Autodesk Fusion 360 part; units mm, degrees
note: some values were not read from the file. Chosen so that the rebuilt part matches the saved one: which pieces of a blend or face edit are solid. Set by a fixed rule: which sketch regions a step uses.
(part 3 of 3)
  spline S271 degree 3 poles (76.9459, -1.2857) (76.9874, -1.1697) (77.0261, -1.0528) (77.0796, -0.8969) knots 0 0 0 0 1 1 1 1
  line L24 (77.0796, -0.8969) -> (71.8772, -0.8969)
  spline S272 degree 3 poles (71.8772, -0.8969) (71.8728, -0.8474) (71.8656, -0.8253) (71.87, -0.8059) knots 0 0 0 0 1 1 1 1
  spline S273 degree 2 poles (71.87, -0.8059) (72.0386, -0.0634) (72.7928, -0.0634) knots 0 0 0 1 1 1
  spline S274 degree 3 poles (72.7928, -0.0634) (75.5433, -0.0634) (78.2938, -0.0634) (81.0442, -0.0634) knots 0 0 0 0 1 1 1 1
  line L25 (81.0442, -0.0634) -> (81.4689, -0.0634)
  spline S275 degree 3 poles (81.4689, -0.0634) (81.3172, -0.5003) (81.1791, -0.9064) (81.0355, -1.3105) knots 0 0 0 0 1 1 1 1
  spline S276 degree 3 poles (81.0355, -1.3105) (76.5089, -14.0458) (71.9791, -26.78) (67.4605, -39.5181) knots 0 0 0 0 1 1 1 1
  spline S277 degree 3 poles (67.4605, -39.5181) (67.1403, -40.4209) (66.8922, -41.3499) (66.6319, -42.2727) knots 0 0 0 0 1 1 1 1
  spline S278 degree 3 poles (66.6319, -42.2727) (66.5643, -42.5124) (66.5592, -42.7745) (66.5563, -43.0267) knots 0 0 0 0 1 1 1 1
  spline S279 degree 3 poles (66.5563, -43.0267) (66.5417, -44.2641) (67.3792, -44.9721) (68.5993, -44.764) knots 0 0 0 0 1 1 1 1
  spline S280 degree 3 poles (68.5993, -44.764) (69.1748, -44.6659) (69.6796, -44.4126) (70.1463, -44.0705) knots 0 0 0 0 1 1 1 1
  spline S281 degree 3 poles (70.1463, -44.0705) (71.6905, -42.9385) (72.8455, -41.4761) (73.6418, -39.7556) knots 0 0 0 0 1 1 1 1
  spline S282 degree 3 poles (73.6418, -39.7556) (74.1085, -38.7475) (74.4293, -37.6709) (74.7999, -36.6195) knots 0 0 0 0 1 1 1 1
  spline S283 degree 3 poles (74.7999, -36.6195) (76.6624, -31.3356) (78.5196, -26.0499) (80.3787, -20.7648) knots 0 0 0 0 1 1 1 1
  spline S284 degree 3 poles (80.3787, -20.7648) (80.4133, -20.6665) (80.4479, -20.5681) (80.4962, -20.4306) knots 0 0 0 0 1 1 1 1
  line L26 (80.4962, -20.4306) -> (75.2552, -20.4306)
  spline S285 degree 3 poles (75.2552, -20.4306) (75.3359, -20.148) (75.3825, -19.9022) (75.4831, -19.6808) knots 0 0 0 0 1 1 1 1
  spline S286 degree 3 poles (75.4831, -19.6808) (75.5151, -19.6102) (75.6902, -19.574) (75.8, -19.5737) knots 0 0 0 0 1 1 1 1
  spline S287 degree 3 poles (75.8, -19.5737) (77.8099, -19.5675) (79.8199, -19.5691) (81.8299, -19.5691) knots 0 0 0 0 1 1 1 1
  spline S288 degree 3 poles (81.8299, -19.5691) (82.7185, -19.5691) (83.6071, -19.5691) (84.4957, -19.5691) knots 0 0 0 0 1 1 1 1
  line L27 (84.4957, -19.5691) -> (84.8908, -19.5691)
  spline S289 degree 3 poles (84.8908, -19.5691) (84.6969, -20.1342) (84.5194, -20.6587) (84.3372, -21.1815) knots 0 0 0 0 1 1 1 1
  spline S290 degree 3 poles (84.3372, -21.1815) (82.1946, -27.3287) (80.0448, -33.4733) (77.9153, -39.625) knots 0 0 0 0 1 1 1 1
  spline S291 degree 3 poles (77.9153, -39.625) (77.5918, -40.5594) (77.343, -41.5214) (77.099, -42.4806) knots 0 0 0 0 1 1 1 1
  spline S292 degree 3 poles (77.099, -42.4806) (77.0232, -42.7789) (77.0352, -43.1161) (77.0794, -43.4251) knots 0 0 0 0 1 1 1 1
  spline S293 degree 3 poles (77.0794, -43.4251) (77.2211, -44.4149) (78.0389, -44.9766) (79.081, -44.7494) knots 0 0 0 0 1 1 1 1
  spline S294 degree 3 poles (79.081, -44.7494) (79.5647, -44.644) (80.0606, -44.4492) (80.4698, -44.1743) knots 0 0 0 0 1 1 1 1
  spline S295 degree 3 poles (80.4698, -44.1743) (81.9568, -43.1756) (83.0471, -41.8112) (83.893, -40.2456) knots 0 0 0 0 1 1 1 1
  spline S296 degree 3 poles (83.893, -40.2456) (83.9344, -40.169) (83.9365, -40.0409) (83.9031, -39.9585) knots 0 0 0 0 1 1 1 1
  spline S297 degree 3 poles (83.9031, -39.9585) (82.6174, -36.7855) (82.7766, -33.5787) (83.9322, -30.4535) knots 0 0 0 0 1 1 1 1
  spline S298 degree 3 poles (83.9322, -30.4535) (85.9017, -25.1273) (89.5691, -21.403) (94.9427, -19.4482) knots 0 0 0 0 1 1 1 1
  spline S299 degree 3 poles (94.9427, -19.4482) (96.8678, -18.7478) (98.865, -18.5551) (100.8691, -19.0689) knots 0 0 0 0 1 1 1 1
  spline S300 degree 3 poles (100.8691, -19.0689) (103.3851, -19.714) (105.1687, -21.313) (106.3628, -23.5722) knots 0 0 0 0 1 1 1 1
  spline S301 degree 3 poles (106.3628, -23.5722) (107.5188, -25.7593) (107.8486, -28.1077) (107.5537, -30.5511) knots 0 0 0 0 1 1 1 1
  spline S302 degree 3 poles (107.5537, -30.5511) (107.0753, -34.5158) (105.1593, -37.7643) (102.4686, -40.6044) knots 0 0 0 0 1 1 1 1
  spline S303 degree 3 poles (102.4686, -40.6044) (100.6012, -42.5754) (98.3827, -44.0429) (95.8081, -44.9372) knots 0 0 0 0 1 1 1 1
  spline S304 degree 3 poles (95.8081, -44.9372) (93.5986, -45.7048) (91.3614, -45.8636) (89.1334, -45.0354) knots 0 0 0 0 1 1 1 1
  spline S305 degree 3 poles (89.1334, -45.0354) (87.2073, -44.3196) (85.7144, -43.047) (84.6127, -41.3152) knots 0 0 0 0 1 1 1 1
  spline S306 degree 3 poles (84.6127, -41.3152) (84.5617, -41.2351) (84.5132, -41.1534) (84.4605, -41.0746) knots 0 0 0 0 1 1 1 1
  spline S307 degree 3 poles (84.4605, -41.0746) (84.4504, -41.0594) (84.4258, -41.054) (84.4744, -41.0809) knots 0 0 0 0 1 1 1 1
  spline S308 degree 3 poles (84.4744, -41.0809) (83.8997, -41.8316) (83.3916, -42.6279) (82.7546, -43.3024) knots 0 0 0 0 1 1 1 1
  spline S309 degree 3 poles (82.7546, -43.3024) (80.844, -45.3252) (78.4925, -45.9992) (75.7898, -45.3455) knots 0 0 0 0 1 1 1 1
  spline S310 degree 3 poles (75.7898, -45.3455) (74.2035, -44.9618) (73.427, -43.9443) (73.377, -42.3173) knots 0 0 0 0 1 1 1 1
  spline S311 degree 3 poles (73.377, -42.3173) (73.3743, -42.2262) (73.3767, -42.1348) (73.3767, -41.9795) knots 0 0 0 0 1 1 1 1
  spline S312 degree 3 poles (73.3767, -41.9795) (73.0458, -42.3875) (72.7758, -42.7603) (72.4656, -43.096) knots 0 0 0 0 1 1 1 1
  spline S313 degree 3 poles (72.4656, -43.096) (71.2784, -44.3806) (69.8832, -45.31) (68.0996, -45.5148) knots 0 0 0 0 1 1 1 1
  spline S314 degree 3 poles (68.0996, -45.5148) (67.0306, -45.6375) (65.9669, -45.6042) (64.9382, -45.2356) knots 0 0 0 0 1 1 1 1
  spline S315 degree 3 poles (64.9382, -45.2356) (63.5857, -44.7511) (62.923, -43.8262) (62.8928, -42.3877) knots 0 0 0 0 1 1 1 1
  spline S316 degree 3 poles (62.8928, -42.3877) (62.8902, -42.2662) (62.8925, -42.1445) (62.8925, -41.9728) knots 0 0 0 0 1 1 1 1
  spline S317 degree 3 poles (62.8925, -41.9728) (62.5336, -42.4076) (62.2327, -42.813) (61.8902, -43.1798) knots 0 0 0 0 1 1 1 1
  spline S318 degree 3 poles (61.8902, -43.1798) (60.4964, -44.6726) (58.821, -45.5971) (56.731, -45.5649) knots 0 0 0 0 1 1 1 1
  spline S319 degree 3 poles (56.731, -45.5649) (56.0409, -45.5543) (55.3375, -45.4608) (54.6679, -45.2941) knots 0 0 0 0 1 1 1 1
  spline S320 degree 3 poles (54.6679, -45.2941) (53.5786, -45.0228) (53.0763, -44.5495) (52.6072, -43.5745) knots 0 0 0 0 1 1 1 1
  spline S321 degree 3 poles (52.6072, -43.5745) (52.0194, -43.9749) (51.4482, -44.4101) (50.8342, -44.773) knots 0 0 0 0 1 1 1 1
  spline S322 degree 3 poles (50.8342, -44.773) (49.3654, -45.6409) (47.775, -45.7703) (46.1469, -45.3786) knots 0 0 0 0 1 1 1 1
  spline S323 degree 3 poles (46.1469, -45.3786) (44.7538, -45.0434) (43.9596, -44.0239) (43.8607, -42.5731) knots 0 0 0 0 1 1 1 1
  spline S324 degree 3 poles (43.8607, -42.5731) (43.7805, -41.3953) (44.0412, -40.2656) (44.3478, -39.1425) knots 0 0 0 0 1 1 1 1
  spline S325 degree 3 poles (44.3478, -39.1425) (44.3802, -39.0239) (44.4122, -38.9052) (44.3822, -38.747) knots 0 0 0 0 1 1 1 1
  spline S326 degree 3 poles (44.3822, -38.747) (44.2975, -38.8447) (44.2114, -38.9412) (44.1283, -39.0402) knots 0 0 0 0 1 1 1 1
  spline S327 degree 3 poles (44.1283, -39.0402) (42.8844, -40.5225) (41.6555, -42.0196) (40.0946, -43.1941) knots 0 0 0 0 1 1 1 1
  spline S328 degree 3 poles (40.0946, -43.1941) (38.6342, -44.293) (37.0632, -45.1607) (35.2298, -45.4504) knots 0 0 0 0 1 1 1 1
  spline S329 degree 3 poles (35.2298, -45.4504) (33.7641, -45.6821) (32.3176, -45.6378) (30.9433, -45.0022) knots 0 0 0 0 1 1 1 1
  spline S330 degree 3 poles (30.9433, -45.0022) (29.1176, -44.1579) (28.0823, -42.6659) (27.6348, -40.7633) knots 0 0 0 0 1 1 1 1
  spline S331 degree 3 poles (27.6348, -40.7633) (27.443, -39.948) (27.4212, -39.0926) (27.3272, -38.2549) knots 0 0 0 0 1 1 1 1
  spline S332 degree 3 poles (27.3272, -38.2549) (27.3127, -38.1253) (27.3252, -37.9926) (27.2528, -37.8437) knots 0 0 0 0 1 1 1 1
  spline S333 degree 3 poles (27.2528, -37.8437) (27.118, -38.0638) (26.9879, -38.287) (26.8476, -38.5034) knots 0 0 0 0 1 1 1 1
  spline S334 degree 3 poles (26.8476, -38.5034) (24.8612, -41.5667) (22.1611, -43.7524) (18.7272, -44.9928) knots 0 0 0 0 1 1 1 1
  spline S335 degree 3 poles (18.7272, -44.9928) (16.8655, -45.6654) (14.9147, -45.7043) (12.9615, -45.5794) knots 0 0 0 0 1 1 1 1
  spline S336 degree 3 poles (12.9615, -45.5794) (11.4556, -45.483) (9.982, -45.2081) (8.5868, -44.6156) knots 0 0 0 0 1 1 1 1
  spline S337 degree 3 poles (8.5868, -44.6156) (5.0699, -43.1219) (2.7269, -40.5128) (1.4018, -36.9651) knots 0 0 0 0 1 1 1 1
  spline S338 degree 3 poles (1.4018, -36.9651) (0.5889, -34.789) (0.2461, -32.5189) (0.1152, -30.2088) knots 0 0 0 0 1 1 1 1
  spline S339 degree 3 poles (0.1152, -30.2088) (-0.1988, -24.667) (1.4603, -19.6798) (4.4487, -15.0988) knots 0 0 0 0 1 1 1 1
  spline S340 degree 3 poles (4.4487, -15.0988) (7.6391, -10.2081) (11.8716, -6.4708) (17.171, -3.9759) knots 0 0 0 0 1 1 1 1
  spline S341 degree 3 poles (17.171, -3.9759) (18.9174, -3.1537) (20.7361, -2.5457) (22.6573, -2.2749) knots 0 0 0 0 1 1 1 1
  spline S342 degree 3 poles (22.6573, -2.2749) (25.2538, -1.9088) (27.7778, -2.2096) (30.2365, -3.0973) knots 0 0 0 0 1 1 1 1
  spline S343 degree 3 poles (30.2365, -3.0973) (31.1101, -3.4127) (31.9675, -3.7753) (32.8488, -4.0666) knots 0 0 0 0 1 1 1 1
  spline S344 degree 3 poles (32.8488, -4.0666) (33.3657, -4.2376) (33.9099, -4.3637) (34.4509, -4.4166) knots 0 0 0 0 1 1 1 1
  spline S345 degree 3 poles (34.4509, -4.4166) (35.5622, -4.5251) (36.3629, -3.9783) (36.9084, -3.0554) knots 0 0 0 0 1 1 1 1
  spline S346 degree 3 poles (36.9084, -3.0554) (37.0752, -2.7732) (37.2322, -2.6868) (37.5281, -2.7909) knots 0 0 0 0 1 1 1 1
  spline S347 degree 3 poles (37.5281, -2.7909) (37.6735, -2.8421) (37.8301, -2.8615) (38.014, -2.9026) knots 0 0 0 0 1 1 1 1
  spline S348 degree 3 poles (38.014, -2.9026) (37.7215, -3.721) (37.4387, -4.513) (37.1555, -5.3048) knots 0 0 0 0 1 1 1 1
  spline S349 degree 3 poles (37.1555, -5.3048) (36.1535, -8.1065) (35.1509, -10.908) (34.1497, -13.71) knots 0 0 0 0 1 1 1 1
  spline S350 degree 3 poles (34.1497, -13.71) (33.9218, -14.3478) (33.924, -14.3486) (33.1894, -14.2539) knots 0 0 0 0 1 1 1 1
  spline S351 degree 3 poles (33.1894, -14.2539) (33.2661, -13.6185) (33.3592, -12.9843) (33.4161, -12.3467) knots 0 0 0 0 1 1 1 1
  spline S352 degree 3 poles (33.4161, -12.3467) (33.5354, -11.0084) (33.6343, -9.6642) (33.2979, -8.3429) knots 0 0 0 0 1 1 1 1
  spline S353 degree 3 poles (33.2979, -8.3429) (32.7503, -6.1919) (31.4072, -4.6744) (29.3636, -3.8873) knots 0 0 0 0 1 1 1 1
  spline S354 degree 3 poles (29.3636, -3.8873) (25.4024, -2.3618) (21.6115, -2.5974) (18.1064, -5.2075) knots 0 0 0 0 1 1 1 1
  spline S355 degree 3 poles (18.1064, -5.2075) (15.5983, -7.0752) (13.6497, -9.4342) (12.0128, -12.064) knots 0 0 0 0 1 1 1 1
  spline S356 degree 3 poles (12.0128, -12.064) (9.4965, -16.1067) (7.7161, -20.4766) (6.3534, -25.0241) knots 0 0 0 0 1 1 1 1
  spline S357 degree 3 poles (6.3534, -25.0241) (5.5761, -27.6183) (5.0135, -30.2599) (4.7229, -32.9543) knots 0 0 0 0 1 1 1 1
  spline S358 degree 3 poles (4.7229, -32.9543) (4.5192, -34.842) (4.4781, -36.7259) (4.9304, -38.5933) knots 0 0 0 0 1 1 1 1
  spline S359 degree 3 poles (4.9304, -38.5933) (5.6053, -41.3794) (7.3021, -43.2695) (10.0108, -44.1478) knots 0 0 0 0 1 1 1 1
  spline S360 degree 3 poles (10.0108, -44.1478) (13.1649, -45.1705) (16.3359, -45.2186) (19.4152, -43.8207) knots 0 0 0 0 1 1 1 1
  spline S361 degree 3 poles (19.4152, -43.8207) (22.1935, -42.5594) (24.3784, -40.5957) (26.0144, -38.024) knots 0 0 0 0 1 1 1 1
  spline S362 degree 3 poles (26.0144, -38.024) (26.4452, -37.3469) (26.7981, -36.6105) (27.2978, -35.9909) knots 0 0 0 0 1 1 1 1
  spline S363 degree 3 poles (27.2978, -35.9909) (27.6013, -35.6146) (27.6548, -35.2071) (27.7761, -34.8009) knots 0 0 0 0 1 1 1 1
  spline S364 degree 3 poles (27.7761, -34.8009) (28.5607, -32.172) (29.8681, -29.8167) (31.5841, -27.6967) knots 0 0 0 0 1 1 1 1
  spline S365 degree 3 poles (31.5841, -27.6967) (34.2471, -24.4068) (37.4617, -21.785) (41.2974, -19.9603) knots 0 0 0 0 1 1 1 1
  spline S366 degree 3 poles (41.2974, -19.9603) (42.5718, -19.3541) (43.9034, -18.9073) (45.3289, -18.8182) knots 0 0 0 0 1 1 1 1
  spline S367 degree 3 poles (45.3289, -18.8182) (46.5961, -18.7389) (47.768, -19.0007) (48.7702, -19.8267) knots 0 0 0 0 1 1 1 1
  spline S368 degree 3 poles (48.7702, -19.8267) (49.4912, -20.4209) (49.8984, -21.1818) (49.9641, -22.1189) knots 0 0 0 0 1 1 1 1
  spline S369 degree 3 poles (49.9641, -22.1189) (49.9692, -22.1925) (49.9778, -22.2661) (49.9884, -22.3391) knots 0 0 0 0 1 1 1 1
  spline S370 degree 3 poles (49.9884, -22.3391) (49.9927, -22.3689) (50.0063, -22.3974) (50.0157, -22.4264) knots 0 0 0 0 1 1 1 1
  spline S371 degree 3 poles (50.0157, -22.4264) (50.0388, -22.4327) (50.0618, -22.439) (50.0849, -22.4264) knots 0 0 0 0 1 1 1 1
  spline S372 degree 3 poles (103.7652, -25.3114) (103.6868, -24.832) (103.6099, -23.932) (103.3842, -23.071) knots 0 0 0 0 1 1 1 1
  spline S373 degree 3 poles (103.3842, -23.071) (102.9323, -21.3472) (101.8898, -20.1667) (100.0685, -19.7927) knots 0 0 0 0 1 1 1 1
  spline S374 degree 3 poles (100.0685, -19.7927) (97.9906, -19.366) (96.1141, -19.7496) (94.434, -21.0869) knots 0 0 0 0 1 1 1 1
  spline S375 degree 3 poles (94.434, -21.0869) (92.8843, -22.3203) (91.7133, -23.8561) (90.75, -25.561) knots 0 0 0 0 1 1 1 1
  spline S376 degree 3 poles (90.75, -25.561) (88.9387, -28.7669) (87.8127, -32.2136) (87.2249, -35.8387) knots 0 0 0 0 1 1 1 1
  spline S377 degree 3 poles (87.2249, -35.8387) (86.9707, -37.4063) (86.8196, -38.9843) (87.089, -40.569) knots 0 0 0 0 1 1 1 1
  spline S378 degree 3 poles (87.089, -40.569) (87.4308, -42.5797) (88.511, -43.9928) (90.5089, -44.5579) knots 0 0 0 0 1 1 1 1
  spline S379 degree 3 poles (90.5089, -44.5579) (92.2381, -45.047) (93.88, -44.7412) (95.3927, -43.7705) knots 0 0 0 0 1 1 1 1
  spline S380 degree 3 poles (95.3927, -43.7705) (96.8708, -42.822) (98.0012, -41.534) (98.9616, -40.0853) knots 0 0 0 0 1 1 1 1
  spline S381 degree 3 poles (98.9616, -40.0853) (100.7237, -37.4275) (101.8987, -34.5089) (102.7607, -31.4561) knots 0 0 0 0 1 1 1 1
  spline S382 degree 3 poles (102.7607, -31.4561) (103.2897, -29.5826) (103.6858, -27.6833) (103.7652, -25.3114) knots 0 0 0 0 1 1 1 1
  spline S383 degree 3 poles (46.0065, -19.6332) (44.9669, -19.627) (44.0162, -19.8508) (43.1126, -20.2652) knots 0 0 0 0 1 1 1 1
  spline S384 degree 3 poles (43.1126, -20.2652) (41.2513, -21.1186) (39.7466, -22.4329) (38.4102, -23.9545) knots 0 0 0 0 1 1 1 1
  spline S385 degree 3 poles (38.4102, -23.9545) (36.618, -25.9951) (35.2451, -28.3068) (34.0956, -30.753) knots 0 0 0 0 1 1 1 1
  spline S386 degree 3 poles (34.0956, -30.753) (32.774, -33.5658) (31.7466, -36.4734) (31.4534, -39.5941) knots 0 0 0 0 1 1 1 1
  spline S387 degree 3 poles (31.4534, -39.5941) (31.3429, -40.7711) (31.3958, -41.9355) (31.8603, -43.0504) knots 0 0 0 0 1 1 1 1
  spline S388 degree 3 poles (31.8603, -43.0504) (32.3368, -44.1941) (33.2068, -44.7345) (34.4271, -44.7672) knots 0 0 0 0 1 1 1 1
  spline S389 degree 3 poles (34.4271, -44.7672) (35.6477, -44.7998) (36.7623, -44.4442) (37.8098, -43.852) knots 0 0 0 0 1 1 1 1
  spline S390 degree 3 poles (37.8098, -43.852) (40.0373, -42.5928) (41.8175, -40.8319) (43.3761, -38.8332) knots 0 0 0 0 1 1 1 1
  spline S391 degree 3 poles (43.3761, -38.8332) (44.1228, -37.8756) (44.8434, -36.8973) (45.2618, -35.7354) knots 0 0 0 0 1 1 1 1
  spline S392 degree 3 poles (45.2618, -35.7354) (46.3267, -32.778) (47.4017, -29.8244) (48.4649, -26.8664) knots 0 0 0 0 1 1 1 1
  spline S393 degree 3 poles (48.4649, -26.8664) (48.8497, -25.7959) (49.3037, -24.7413) (49.4107, -23.5928) knots 0 0 0 0 1 1 1 1
  spline S394 degree 3 poles (49.4107, -23.5928) (49.6232, -21.3105) (48.1691, -19.514) (46.0065, -19.6332) knots 0 0 0 0 1 1 1 1
  spline S395 degree 3 poles (84.1667, -10.1913) (84.1729, -8.6259) (85.3768, -7.4326) (86.9503, -7.4324) knots 0 0 0 0 1 1 1 1
  spline S396 degree 3 poles (86.9503, -7.4324) (88.5314, -7.4321) (89.7239, -8.6369) (89.7211, -10.2316) knots 0 0 0 0 1 1 1 1
  spline S397 degree 3 poles (89.7211, -10.2316) (89.7183, -11.8206) (88.5136, -13.0149) (86.9258, -13.0029) knots 0 0 0 0 1 1 1 1
  spline S398 degree 3 poles (86.9258, -13.0029) (85.3374, -12.9908) (84.1605, -11.7915) (84.1667, -10.1913) knots 0 0 0 0 1 1 1 1
  spline S399 degree 3 poles (128.8614, -26.1716) (128.8153, -28.284) (128.276, -30.6235) (127.5153, -32.9166) knots 0 0 0 0 1 1 1 1
  spline S400 degree 3 poles (127.5153, -32.9166) (126.5931, -35.6965) (125.3817, -38.3368) (123.61, -40.6911) knots 0 0 0 0 1 1 1 1
  spline S401 degree 3 poles (123.61, -40.6911) (122.5647, -42.0801) (121.3489, -43.2903) (119.806, -44.129) knots 0 0 0 0 1 1 1 1
  spline S402 degree 3 poles (119.806, -44.129) (118.0331, -45.0928) (115.4801, -45.0947) (113.845, -43.5861) knots 0 0 0 0 1 1 1 1
  spline S403 degree 3 poles (113.845, -43.5861) (112.9324, -42.7442) (112.3341, -41.7221) (111.9863, -40.5443) knots 0 0 0 0 1 1 1 1
  spline S404 degree 3 poles (111.9863, -40.5443) (111.834, -40.0287) (111.687, -39.5095) (111.5818, -38.983) knots 0 0 0 0 1 1 1 1
  spline S405 degree 3 poles (111.5818, -38.983) (111.5353, -38.7499) (111.5424, -38.4751) (111.6206, -38.2527) knots 0 0 0 0 1 1 1 1
  spline S406 degree 3 poles (111.6206, -38.2527) (113.0797, -34.1034) (114.5515, -29.9585) (116.0281, -25.8153) knots 0 0 0 0 1 1 1 1
  spline S407 degree 3 poles (116.0281, -25.8153) (116.1079, -25.5914) (116.2291, -25.3728) (116.3717, -25.182) knots 0 0 0 0 1 1 1 1
  spline S408 degree 3 poles (116.3717, -25.182) (117.2705, -23.9794) (118.185, -22.7878) (119.3159, -21.7871) knots 0 0 0 0 1 1 1 1
  spline S409 degree 3 poles (119.3159, -21.7871) (120.4047, -20.8235) (121.5941, -20.0336) (123.056, -19.7578) knots 0 0 0 0 1 1 1 1
  spline S410 degree 3 poles (123.056, -19.7578) (123.9276, -19.5934) (124.8028, -19.5937) (125.6676, -19.8061) knots 0 0 0 0 1 1 1 1
  spline S411 degree 3 poles (125.6676, -19.8061) (126.9085, -20.111) (127.6838, -20.9266) (128.1613, -22.0809) knots 0 0 0 0 1 1 1 1
  spline S412 degree 3 poles (128.1613, -22.0809) (128.6621, -23.2915) (128.8638, -24.5521) (128.8614, -26.1716) knots 0 0 0 0 1 1 1 1
  spline S413 degree 3 poles (138.7712, -30.0038) (139.2283, -29.0291) (139.6235, -28.0968) (140.0927, -27.2034) knots 0 0 0 0 1 1 1 1
  spline S414 degree 3 poles (140.0927, -27.2034) (141.2378, -25.0227) (142.6739, -23.0631) (144.619, -21.5155) knots 0 0 0 0 1 1 1 1
  spline S415 degree 3 poles (144.619, -21.5155) (145.6449, -20.6992) (146.7387, -19.9808) (148.0608, -19.7806) knots 0 0 0 0 1 1 1 1
  spline S416 degree 3 poles (148.0608, -19.7806) (148.7512, -19.6761) (149.4761, -19.6581) (150.1687, -19.7408) knots 0 0 0 0 1 1 1 1
  spline S417 degree 3 poles (150.1687, -19.7408) (151.3327, -19.8797) (152.1161, -20.7367) (152.2726, -21.9102) knots 0 0 0 0 1 1 1 1
  spline S418 degree 3 poles (152.2726, -21.9102) (152.4727, -23.4101) (151.9809, -24.7224) (151.122, -25.9174) knots 0 0 0 0 1 1 1 1
  spline S419 degree 3 poles (151.122, -25.9174) (149.935, -27.569) (148.2949, -28.6145) (146.4395, -29.3662) knots 0 0 0 0 1 1 1 1
  spline S420 degree 3 poles (146.4395, -29.3662) (144.4026, -30.1915) (142.2832, -30.356) (140.1191, -30.1628) knots 0 0 0 0 1 1 1 1
  spline S421 degree 3 poles (140.1191, -30.1628) (139.7002, -30.1254) (139.2833, -30.0649) (138.7712, -30.0038) knots 0 0 0 0 1 1 1 1
  spline S422 degree 3 poles (103.7652, -25.3302) (103.6859, -27.7021) (103.2897, -29.6014) (102.7607, -31.4749) knots 0 0 0 0 1 1 1 1
  spline S423 degree 3 poles (102.7607, -31.4749) (101.8987, -34.5277) (100.7238, -37.4463) (98.9617, -40.1041) knots 0 0 0 0 1 1 1 1
  spline S424 degree 3 poles (98.9617, -40.1041) (98.0012, -41.5528) (96.8709, -42.8408) (95.3927, -43.7893) knots 0 0 0 0 1 1 1 1
  spline S425 degree 3 poles (95.3927, -43.7893) (93.8801, -44.76) (92.2382, -45.0658) (90.509, -44.5767) knots 0 0 0 0 1 1 1 1
  spline S426 degree 3 poles (90.509, -44.5767) (88.511, -44.0116) (87.4309, -42.5985) (87.089, -40.5878) knots 0 0 0 0 1 1 1 1
  spline S427 degree 3 poles (87.089, -40.5878) (86.8196, -39.0031) (86.9707, -37.4251) (87.2249, -35.8575) knots 0 0 0 0 1 1 1 1
  spline S428 degree 3 poles (87.2249, -35.8575) (87.8128, -32.2324) (88.9387, -28.7857) (90.7501, -25.5798) knots 0 0 0 0 1 1 1 1
  spline S429 degree 3 poles (90.7501, -25.5798) (91.7133, -23.8749) (92.8844, -22.3391) (94.4341, -21.1057) knots 0 0 0 0 1 1 1 1
  spline S430 degree 3 poles (94.4341, -21.1057) (96.1142, -19.7684) (97.9907, -19.3848) (100.0686, -19.8115) knots 0 0 0 0 1 1 1 1
  spline S431 degree 3 poles (100.0686, -19.8115) (101.8899, -20.1855) (102.9323, -21.366) (103.3842, -23.0898) knots 0 0 0 0 1 1 1 1
  spline S432 degree 3 poles (103.3842, -23.0898) (103.61, -23.9508) (103.6869, -24.8508) (103.7652, -25.3302) knots 0 0 0 0 1 1 1 1
  spline S433 degree 3 poles (46.0066, -19.652) (48.1692, -19.5328) (49.6232, -21.3293) (49.4107, -23.6116) knots 0 0 0 0 1 1 1 1
  spline S434 degree 3 poles (49.4107, -23.6116) (49.3038, -24.7601) (48.8497, -25.8147) (48.4649, -26.8852) knots 0 0 0 0 1 1 1 1
  spline S435 degree 3 poles (48.4649, -26.8852) (47.4017, -29.8432) (46.3267, -32.7968) (45.2618, -35.7542) knots 0 0 0 0 1 1 1 1
  spline S436 degree 3 poles (45.2618, -35.7542) (44.8434, -36.9161) (44.1228, -37.8944) (43.3761, -38.852) knots 0 0 0 0 1 1 1 1
  spline S437 degree 3 poles (43.3761, -38.852) (41.8175, -40.8507) (40.0373, -42.6116) (37.8099, -43.8708) knots 0 0 0 0 1 1 1 1
  spline S438 degree 3 poles (37.8099, -43.8708) (36.7624, -44.463) (35.6477, -44.8186) (34.4271, -44.786) knots 0 0 0 0 1 1 1 1
  spline S439 degree 3 poles (34.4271, -44.786) (33.2068, -44.7533) (32.3368, -44.213) (31.8603, -43.0692) knots 0 0 0 0 1 1 1 1
  spline S440 degree 3 poles (31.8603, -43.0692) (31.3958, -41.9543) (31.3429, -40.7899) (31.4535, -39.6129) knots 0 0 0 0 1 1 1 1
  spline S441 degree 3 poles (31.4535, -39.6129) (31.7466, -36.4922) (32.774, -33.5846) (34.0957, -30.7718) knots 0 0 0 0 1 1 1 1
  spline S442 degree 3 poles (34.0957, -30.7718) (35.2451, -28.3256) (36.618, -26.0139) (38.4102, -23.9733) knots 0 0 0 0 1 1 1 1
  spline S443 degree 3 poles (38.4102, -23.9733) (39.7466, -22.4517) (41.2513, -21.1374) (43.1126, -20.284) knots 0 0 0 0 1 1 1 1
  spline S444 degree 3 poles (43.1126, -20.284) (44.0162, -19.8697) (44.967, -19.6458) (46.0066, -19.652) knots 0 0 0 0 1 1 1 1
  line L28 (156.0195, -22.8998) -> (156.0195, -23.5976)
extrude "Extrude1" [suppressed]
extrude "Extrude2" [suppressed]
sketch "Sketch2" plane through (0, 0, 0) normal (0, 0, 1) x (1, 0, 0)
  line L0 (155.956, -22.86) -> (155.956, -23.876)
  constraint vertical L0
